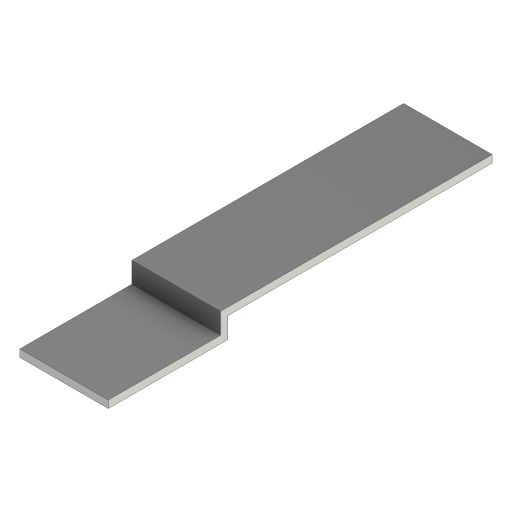
# Autodesk Inventor part: shelf
Saved by Autodesk Inventor 2023 (Build 270158000, 158)
## iProperties
Created: 2022-09-12
Part Number: shelf
Material: 常规
Document SubType Name: Modeling
Designer: byfbi
Density: 1 g/cm^3
Appearance: 默认
Author: byfbi
Autodesk Inventor part; units mm, degrees
ref_plane "YZ Plane" through (0, 0, 0) normal (1, 0, 0) x (0, 1, 0)
ref_plane "XZ Plane" through (0, 0, 0) normal (0, 1, 0) x (-1, 0, 0)
sketch "草图1" plane through (0, 0, 0) normal (1, 0, 0) x (0, 1, 0)
  line L0 (0, 0) -> (0, -810)
  line L1 (0, -810) -> (140, -810)
  line L2 (140, -810) -> (140, -2600)
  line L3 (190, -2600) -> (190, -760)
  line L4 (190, -760) -> (50, -760)
  line L5 (50, -760) -> (50, 0)
  line L6 (50, 0) -> (0, 0)
  line L7 (190, -2600) -> (140, -2600)
  dimension "d0" = 810
  dimension "d1" = 140
  dimension "d2" = 2600
  dimension "d3" = 50
  constraints: 16 end point, 4 perpendicular, 1 horizontal, 1 parallel, 1 vertical, 2 other
  measures "d0" distance of L0.start L0.end
  measures "d1" distance of L0.end L1.end
  measures "d2" vertical distance of L2.end L0.start
  measures "d3" distance between parallel lines of L2 L3
extrude "拉伸1" add sketch "草图1" along normal blind 600
ref_plane "工作平面1" through (0, 690, -760) normal (0, 1, 0) x (1, 0, 0)
